Autodesk Fusion 360 part; units mm, degrees
note: some values were not read from the file. Chosen so that the rebuilt part matches the saved one: a direction. Set by a fixed rule: which sketch regions a step uses.
(part 2 of 5)
  arc A27 (-12.0685, 25.5855) -> (-12.156, 25.4753) centre (-12.0566, 25.4862) ccw
  arc A28 (-12.0685, 25.5855) -> (-11.0585, 25.7494) centre (-13.5, 37.5997) ccw
  arc A29 (-10.9406, 25.6726) -> (-11.0585, 25.7494) centre (-11.0383, 25.6515) ccw
  line L14 (-10.9406, 25.6726) -> (-10.8377, 25.1964)
  spline S14 degree 5 poles (-10.8377, 25.1964) (-10.8365, 25.1908) (-10.834, 25.1798) (-10.8298, 25.1634) (-10.8235, 25.1417) (-10.8145, 25.1148) (-10.8047, 25.0882) (-10.7944, 25.0617) (-10.7839, 25.0352) (-10.7732, 25.0088) (-10.7623, 24.9824) (-10.7512, 24.9561) (-10.7398, 24.9298) (-10.7279, 24.9037) (-10.7158, 24.8777) (-10.7032, 24.8517) (-10.6904, 24.8259) (-10.6773, 24.8001) (-10.664, 24.7744) (-10.6505, 24.7488) (-10.6368, 24.7232) (-10.6229, 24.6977) (-10.6088, 24.6723) (-10.5944, 24.6469) (-10.5798, 24.6216) (-10.565, 24.5964) (-10.55, 24.5712) (-10.5348, 24.5461) (-10.5194, 24.5211) (-10.5038, 24.4961) (-10.488, 24.4712) (-10.472, 24.4464) (-10.4558, 24.4216) (-10.4395, 24.3969) (-10.423, 24.3722) (-10.4063, 24.3476) (-10.3894, 24.3231) (-10.3724, 24.2987) (-10.3551, 24.2743) (-10.3378, 24.2499) (-10.3202, 24.2257) (-10.3025, 24.2015) (-10.2846, 24.1773) (-10.2666, 24.1533) (-10.2484, 24.1292) (-10.2301, 24.1053) (-10.2116, 24.0814) (-10.1929, 24.0576) (-10.1741, 24.0338) (-10.1551, 24.0101) (-10.136, 23.9865) (-10.1167, 23.9629) (-10.0973, 23.9394) (-10.0778, 23.9159) (-10.0581, 23.8925) (-10.0382, 23.8692) (-10.0183, 23.846) (-9.9981, 23.8228) (-9.9779, 23.7996) (-9.9575, 23.7766) (-9.9369, 23.7535) (-9.9162, 23.7306) (-9.8954, 23.7077) (-9.8745, 23.6849) (-9.8534, 23.6621) (-9.8322, 23.6395) (-9.8108, 23.6168) (-9.7893, 23.5943) (-9.7677, 23.5718) (-9.746, 23.5493) (-9.7241, 23.527) (-9.7065, 23.5091) (-9.6932, 23.4958) (-9.6844, 23.4869) (-9.6799, 23.4824) knots 0 0 0 0 0 0 0.01428571 0.02857143 0.04285714 0.05714286 0.07142857 0.08571429 0.1 0.11428571 0.12857143 0.14285714 0.15714286 0.17142857 0.18571429 0.2 0.21428571 0.22857143 0.24285714 0.25714286 0.27142857 0.28571429 0.3 0.31428571 0.32857143 0.34285714 0.35714286 0.37142857 0.38571429 0.4 0.41428571 0.42857143 0.44285714 0.45714286 0.47142857 0.48571429 0.5 0.51428571 0.52857143 0.54285714 0.55714286 0.57142857 0.58571429 0.6 0.61428571 0.62857143 0.64285714 0.65714286 0.67142857 0.68571429 0.7 0.71428571 0.72857143 0.74285714 0.75714286 0.77142857 0.78571429 0.8 0.81428571 0.82857143 0.84285714 0.85714286 0.87142857 0.88571429 0.9 0.91428571 0.92857143 0.94285714 0.95714286 0.97142857 0.98571429 1 1 1 1 1 1
  arc A30 (-9.6799, 23.4824) -> (-8.909, 23.714) centre (-13.5, 37.5997) ccw
  spline S15 degree 5 poles (-8.909, 23.714) (-8.9078, 23.7201) (-8.9053, 23.7324) (-8.9016, 23.7509) (-8.8967, 23.7755) (-8.8908, 23.8062) (-8.885, 23.8369) (-8.8794, 23.8676) (-8.8739, 23.8982) (-8.8685, 23.9289) (-8.8633, 23.9595) (-8.8583, 23.9901) (-8.8533, 24.0207) (-8.8486, 24.0513) (-8.844, 24.0818) (-8.8395, 24.1123) (-8.8352, 24.1428) (-8.831, 24.1733) (-8.827, 24.2038) (-8.8231, 24.2342) (-8.8194, 24.2646) (-8.8159, 24.295) (-8.8125, 24.3253) (-8.8092, 24.3556) (-8.8062, 24.3859) (-8.8032, 24.4162) (-8.8005, 24.4464) (-8.7979, 24.4766) (-8.7954, 24.5068) (-8.7931, 24.5369) (-8.791, 24.567) (-8.7891, 24.597) (-8.7873, 24.6271) (-8.7857, 24.6571) (-8.7842, 24.687) (-8.783, 24.7169) (-8.7819, 24.7468) (-8.7809, 24.7767) (-8.7802, 24.8065) (-8.7796, 24.8362) (-8.7792, 24.8659) (-8.779, 24.8956) (-8.779, 24.9252) (-8.7792, 24.9548) (-8.7795, 24.9843) (-8.7801, 25.0138) (-8.7808, 25.0433) (-8.7818, 25.0726) (-8.7829, 25.102) (-8.7842, 25.1312) (-8.7857, 25.1605) (-8.7875, 25.1896) (-8.7895, 25.2187) (-8.7917, 25.2477) (-8.7942, 25.2767) (-8.7968, 25.3056) (-8.7997, 25.3344) (-8.8028, 25.3632) (-8.806, 25.3919) (-8.8096, 25.4205) (-8.8134, 25.4491) (-8.8176, 25.4775) (-8.8221, 25.5058) (-8.827, 25.534) (-8.8323, 25.5621) (-8.8377, 25.5901) (-8.8433, 25.6181) (-8.8491, 25.646) (-8.8552, 25.6737) (-8.8617, 25.7014) (-8.869, 25.7287) (-8.8757, 25.7503) (-8.8812, 25.7663) (-8.8852, 25.7769) (-8.8873, 25.7822) knots -1 -1 -1 -1 -1 -1 -0.98571429 -0.97142857 -0.95714286 -0.94285714 -0.92857143 -0.91428571 -0.9 -0.88571429 -0.87142857 -0.85714286 -0.84285714 -0.82857143 -0.81428571 -0.8 -0.78571429 -0.77142857 -0.75714286 -0.74285714 -0.72857143 -0.71428571 -0.7 -0.68571429 -0.67142857 -0.65714286 -0.64285714 -0.62857143 -0.61428571 -0.6 -0.58571429 -0.57142857 -0.55714286 -0.54285714 -0.52857143 -0.51428571 -0.5 -0.48571429 -0.47142857 -0.45714286 -0.44285714 -0.42857143 -0.41428571 -0.4 -0.38571429 -0.37142857 -0.35714286 -0.34285714 -0.32857143 -0.31428571 -0.3 -0.28571429 -0.27142857 -0.25714286 -0.24285714 -0.22857143 -0.21428571 -0.2 -0.18571429 -0.17142857 -0.15714286 -0.14285714 -0.12857143 -0.11428571 -0.1 -0.08571429 -0.07142857 -0.05714286 -0.04285714 -0.02857143 -0.01428571 0 0 0 0 0 0
  line L15 (-8.8873, 25.7822) -> (-9.0638, 26.2363)
  arc A31 (-9.0077, 26.3654) -> (-9.0638, 26.2363) centre (-8.9706, 26.2725) ccw
  arc A32 (-9.0077, 26.3654) -> (-8.0746, 26.7851) centre (-13.5, 37.5997) ccw
  arc A33 (-7.9408, 26.7414) -> (-8.0746, 26.7851) centre (-8.0298, 26.6957) ccw
  line L16 (-7.9408, 26.7414) -> (-7.7182, 26.3081)
  spline S16 degree 5 poles (-7.7182, 26.3081) (-7.7156, 26.303) (-7.7103, 26.293) (-7.702, 26.2782) (-7.6903, 26.2589) (-7.6746, 26.2353) (-7.6583, 26.2121) (-7.6416, 26.1891) (-7.6245, 26.1663) (-7.6074, 26.1435) (-7.59, 26.1209) (-7.5724, 26.0983) (-7.5546, 26.076) (-7.5364, 26.0538) (-7.5179, 26.0318) (-7.4991, 26.01) (-7.48, 25.9883) (-7.4607, 25.9668) (-7.4413, 25.9454) (-7.4216, 25.9242) (-7.4017, 25.903) (-7.3817, 25.882) (-7.3614, 25.861) (-7.341, 25.8403) (-7.3203, 25.8196) (-7.2995, 25.7991) (-7.2785, 25.7786) (-7.2573, 25.7583) (-7.2359, 25.7382) (-7.2144, 25.7181) (-7.1927, 25.6981) (-7.1708, 25.6782) (-7.1488, 25.6585) (-7.1266, 25.6389) (-7.1043, 25.6193) (-7.0818, 25.5999) (-7.0592, 25.5806) (-7.0364, 25.5614) (-7.0134, 25.5423) (-6.9903, 25.5233) (-6.9671, 25.5044) (-6.9437, 25.4856) (-6.9202, 25.4669) (-6.8966, 25.4483) (-6.8728, 25.4298) (-6.8489, 25.4114) (-6.8248, 25.3931) (-6.8006, 25.375) (-6.7763, 25.3569) (-6.7518, 25.3389) (-6.7273, 25.321) (-6.7026, 25.3032) (-6.6777, 25.2855) (-6.6528, 25.2679) (-6.6277, 25.2504) (-6.6025, 25.233) (-6.5772, 25.2157) (-6.5517, 25.1985) (-6.5262, 25.1814) (-6.5005, 25.1644) (-6.4747, 25.1475) (-6.4488, 25.1307) (-6.4227, 25.114) (-6.3966, 25.0974) (-6.3703, 25.0809) (-6.3439, 25.0644) (-6.3175, 25.0481) (-6.2909, 25.0319) (-6.2642, 25.0158) (-6.2374, 24.9997) (-6.2104, 24.9838) (-6.1888, 24.9711) (-6.1726, 24.9616) (-6.1617, 24.9553) (-6.1563, 24.9522) knots 0 0 0 0 0 0 0.01428571 0.02857143 0.04285714 0.05714286 0.07142857 0.08571429 0.1 0.11428571 0.12857143 0.14285714 0.15714286 0.17142857 0.18571429 0.2 0.21428571 0.22857143 0.24285714 0.25714286 0.27142857 0.28571429 0.3 0.31428571 0.32857143 0.34285714 0.35714286 0.37142857 0.38571429 0.4 0.41428571 0.42857143 0.44285714 0.45714286 0.47142857 0.48571429 0.5 0.51428571 0.52857143 0.54285714 0.55714286 0.57142857 0.58571429 0.6 0.61428571 0.62857143 0.64285714 0.65714286 0.67142857 0.68571429 0.7 0.71428571 0.72857143 0.74285714 0.75714286 0.77142857 0.78571429 0.8 0.81428571 0.82857143 0.84285714 0.85714286 0.87142857 0.88571429 0.9 0.91428571 0.92857143 0.94285714 0.95714286 0.97142857 0.98571429 1 1 1 1 1 1
  arc A34 (-6.1563, 24.9522) -> (-5.4716, 25.3754) centre (-13.5, 37.5997) ccw
  spline S17 degree 5 poles (-5.4716, 25.3754) (-5.472, 25.3816) (-5.4727, 25.3942) (-5.4739, 25.4129) (-5.4756, 25.4379) (-5.4778, 25.4691) (-5.4802, 25.5003) (-5.4827, 25.5314) (-5.4853, 25.5624) (-5.4881, 25.5934) (-5.491, 25.6244) (-5.494, 25.6552) (-5.4972, 25.6861) (-5.5005, 25.7168) (-5.5039, 25.7475) (-5.5075, 25.7781) (-5.5112, 25.8087) (-5.5151, 25.8392) (-5.5191, 25.8697) (-5.5232, 25.9001) (-5.5275, 25.9304) (-5.532, 25.9606) (-5.5365, 25.9908) (-5.5412, 26.021) (-5.5461, 26.051) (-5.5511, 26.081) (-5.5563, 26.1109) (-5.5616, 26.1407) (-5.567, 26.1705) (-5.5726, 26.2002) (-5.5784, 26.2298) (-5.5843, 26.2594) (-5.5903, 26.2888) (-5.5965, 26.3182) (-5.6029, 26.3475) (-5.6094, 26.3768) (-5.6161, 26.4059) (-5.6229, 26.435) (-5.6299, 26.464) (-5.637, 26.4929) (-5.6443, 26.5217) (-5.6518, 26.5504) (-5.6595, 26.579) (-5.6673, 26.6075) (-5.6753, 26.6359) (-5.6834, 26.6643) (-5.6918, 26.6925) (-5.7003, 26.7207) (-5.709, 26.7487) (-5.7178, 26.7766) (-5.7269, 26.8045) (-5.7361, 26.8322) (-5.7456, 26.8597) (-5.7552, 26.8872) (-5.7651, 26.9145) (-5.7751, 26.9418) (-5.7854, 26.9689) (-5.7958, 26.9959) (-5.8064, 27.0228) (-5.8172, 27.0495) (-5.8283, 27.0761) (-5.8397, 27.1024) (-5.8514, 27.1286) (-5.8634, 27.1546) (-5.8757, 27.1804) (-5.8883, 27.206) (-5.9009, 27.2316) (-5.9138, 27.257) (-5.9268, 27.2823) (-5.9403, 27.3073) (-5.9544, 27.3318) (-5.9664, 27.3509) (-5.9759, 27.365) (-5.9825, 27.3742) (-5.9858, 27.3787) knots -1 -1 -1 -1 -1 -1 -0.98571429 -0.97142857 -0.95714286 -0.94285714 -0.92857143 -0.91428571 -0.9 -0.88571429 -0.87142857 -0.85714286 -0.84285714 -0.82857143 -0.81428571 -0.8 -0.78571429 -0.77142857 -0.75714286 -0.74285714 -0.72857143 -0.71428571 -0.7 -0.68571429 -0.67142857 -0.65714286 -0.64285714 -0.62857143 -0.61428571 -0.6 -0.58571429 -0.57142857 -0.55714286 -0.54285714 -0.52857143 -0.51428571 -0.5 -0.48571429 -0.47142857 -0.45714286 -0.44285714 -0.42857143 -0.41428571 -0.4 -0.38571429 -0.37142857 -0.35714286 -0.34285714 -0.32857143 -0.31428571 -0.3 -0.28571429 -0.27142857 -0.25714286 -0.24285714 -0.22857143 -0.21428571 -0.2 -0.18571429 -0.17142857 -0.15714286 -0.14285714 -0.12857143 -0.11428571 -0.1 -0.08571429 -0.07142857 -0.05714286 -0.04285714 -0.02857143 -0.01428571 0 0 0 0 0 0
  line L17 (-5.9858, 27.3787) -> (-6.2739, 27.7717)
  arc A35 (-6.2531, 27.9109) -> (-6.2739, 27.7717) centre (-6.1932, 27.8308) ccw
  arc A36 (-6.2531, 27.9109) -> (-5.4605, 28.5578) centre (-13.5, 37.5997) ccw
  arc A37 (-5.3199, 28.5502) -> (-5.4605, 28.5578) centre (-5.394, 28.4831) ccw
  line L18 (-5.3199, 28.5502) -> (-4.9927, 28.1892)
  spline S18 degree 5 poles (-4.9927, 28.1892) (-4.9889, 28.1851) (-4.9812, 28.1768) (-4.9694, 28.1646) (-4.953, 28.149) (-4.9318, 28.1303) (-4.91, 28.1121) (-4.8879, 28.0942) (-4.8656, 28.0766) (-4.8431, 28.059) (-4.8204, 28.0416) (-4.7976, 28.0244) (-4.7746, 28.0074) (-4.7513, 27.9907) (-4.7278, 27.9742) (-4.704, 27.958) (-4.6799, 27.9421) (-4.6557, 27.9263) (-4.6313, 27.9107) (-4.6068, 27.8952) (-4.5822, 27.8799) (-4.5574, 27.8648) (-4.5324, 27.8498) (-4.5073, 27.835) (-4.482, 27.8204) (-4.4565, 27.806) (-4.431, 27.7917) (-4.4052, 27.7776) (-4.3794, 27.7636) (-4.3534, 27.7498) (-4.3272, 27.7361) (-4.301, 27.7226) (-4.2746, 27.7092) (-4.2481, 27.696) (-4.2215, 27.6829) (-4.1947, 27.6699) (-4.1678, 27.6571) (-4.1409, 27.6445) (-4.1138, 27.632) (-4.0865, 27.6196) (-4.0592, 27.6073) (-4.0318, 27.5952) (-4.0042, 27.5833) (-3.9766, 27.5714) (-3.9488, 27.5597) (-3.9209, 27.5482) (-3.893, 27.5367) (-3.8649, 27.5254) (-3.8367, 27.5143) (-3.8084, 27.5032) (-3.7801, 27.4923) (-3.7516, 27.4815) (-3.723, 27.4708) (-3.6944, 27.4603) (-3.6656, 27.4499) (-3.6368, 27.4396) (-3.6078, 27.4295) (-3.5788, 27.4195) (-3.5497, 27.4096) (-3.5205, 27.3998) (-3.4912, 27.3901) (-3.4618, 27.3806) (-3.4323, 27.3712) (-3.4028, 27.3619) (-3.3731, 27.3527) (-3.3434, 27.3437) (-3.3136, 27.3348) (-3.2837, 27.326) (-3.2538, 27.3173) (-3.2237, 27.3088) (-3.1936, 27.3003) (-3.1694, 27.2937) (-3.1513, 27.2887) (-3.1391, 27.2855) (-3.1331, 27.2838) knots 0 0 0 0 0 0 0.01428571 0.02857143 0.04285714 0.05714286 0.07142857 0.08571429 0.1 0.11428571 0.12857143 0.14285714 0.15714286 0.17142857 0.18571429 0.2 0.21428571 0.22857143 0.24285714 0.25714286 0.27142857 0.28571429 0.3 0.31428571 0.32857143 0.34285714 0.35714286 0.37142857 0.38571429 0.4 0.41428571 0.42857143 0.44285714 0.45714286 0.47142857 0.48571429 0.5 0.51428571 0.52857143 0.54285714 0.55714286 0.57142857 0.58571429 0.6 0.61428571 0.62857143 0.64285714 0.65714286 0.67142857 0.68571429 0.7 0.71428571 0.72857143 0.74285714 0.75714286 0.77142857 0.78571429 0.8 0.81428571 0.82857143 0.84285714 0.85714286 0.87142857 0.88571429 0.9 0.91428571 0.92857143 0.94285714 0.95714286 0.97142857 0.98571429 1 1 1 1 1 1
  arc A38 (-3.1331, 27.2838) -> (-2.5812, 27.8698) centre (-13.5, 37.5997) ccw
  spline S19 degree 5 poles (-2.5812, 27.8698) (-2.5832, 27.8757) (-2.5872, 27.8877) (-2.5932, 27.9055) (-2.6013, 27.9292) (-2.6115, 27.9588) (-2.6219, 27.9883) (-2.6323, 28.0177) (-2.6429, 28.047) (-2.6536, 28.0762) (-2.6644, 28.1053) (-2.6753, 28.1343) (-2.6864, 28.1633) (-2.6975, 28.1921) (-2.7088, 28.2209) (-2.7202, 28.2496) (-2.7317, 28.2781) (-2.7433, 28.3066) (-2.7551, 28.335) (-2.767, 28.3633) (-2.7789, 28.3914) (-2.7911, 28.4195) (-2.8033, 28.4475) (-2.8156, 28.4754) (-2.8281, 28.5031) (-2.8407, 28.5308) (-2.8534, 28.5584) (-2.8663, 28.5858) (-2.8792, 28.6132) (-2.8923, 28.6404) (-2.9055, 28.6675) (-2.9189, 28.6945) (-2.9324, 28.7214) (-2.946, 28.7482) (-2.9597, 28.7749) (-2.9735, 28.8014) (-2.9875, 28.8278) (-3.0017, 28.8542) (-3.0159, 28.8803) (-3.0303, 28.9064) (-3.0448, 28.9323) (-3.0595, 28.9581) (-3.0743, 28.9838) (-3.0892, 29.0093) (-3.1043, 29.0347) (-3.1195, 29.06) (-3.1348, 29.0851) (-3.1503, 29.1101) (-3.166, 29.1349) (-3.1818, 29.1596) (-3.1977, 29.1841) (-3.2138, 29.2085) (-3.2301, 29.2327) (-3.2465, 29.2567) (-3.2631, 29.2806) (-3.2799, 29.3043) (-3.2968, 29.3278) (-3.3138, 29.3512) (-3.331, 29.3744) (-3.3484, 29.3974) (-3.366, 29.4202) (-3.3838, 29.4428) (-3.4019, 29.465) (-3.4202, 29.487) (-3.4388, 29.5087) (-3.4575, 29.5303) (-3.4764, 29.5516) (-3.4954, 29.5729) (-3.5145, 29.5939) (-3.534, 29.6146) (-3.554, 29.6346) (-3.5705, 29.65) (-3.5834, 29.6611) (-3.5921, 29.6683) (-3.5965, 29.6718) knots -1 -1 -1 -1 -1 -1 -0.98571429 -0.97142857 -0.95714286 -0.94285714 -0.92857143 -0.91428571 -0.9 -0.88571429 -0.87142857 -0.85714286 -0.84285714 -0.82857143 -0.81428571 -0.8 -0.78571429 -0.77142857 -0.75714286 -0.74285714 -0.72857143 -0.71428571 -0.7 -0.68571429 -0.67142857 -0.65714286 -0.64285714 -0.62857143 -0.61428571 -0.6 -0.58571429 -0.57142857 -0.55714286 -0.54285714 -0.52857143 -0.51428571 -0.5 -0.48571429 -0.47142857 -0.45714286 -0.44285714 -0.42857143 -0.41428571 -0.4 -0.38571429 -0.37142857 -0.35714286 -0.34285714 -0.32857143 -0.31428571 -0.3 -0.28571429 -0.27142857 -0.25714286 -0.24285714 -0.22857143 -0.21428571 -0.2 -0.18571429 -0.17142857 -0.15714286 -0.14285714 -0.12857143 -0.11428571 -0.1 -0.08571429 -0.07142857 -0.05714286 -0.04285714 -0.02857143 -0.01428571 0 0 0 0 0 0
  line L19 (-3.5965, 29.6718) -> (-3.9764, 29.9768)
  arc A39 (-3.9924, 30.1166) -> (-3.9764, 29.9768) centre (-3.9138, 30.0548) ccw
  arc A40 (-3.9924, 30.1166) -> (-3.3942, 30.9467) centre (-13.5, 37.5997) ccw
  arc A41 (-3.2565, 30.9757) -> (-3.3942, 30.9467) centre (-3.3107, 30.8917) ccw
  line L20 (-3.2565, 30.9757) -> (-2.847, 30.7117)
  spline S20 degree 5 poles (-2.847, 30.7117) (-2.8422, 30.7087) (-2.8327, 30.7027) (-2.8181, 30.694) (-2.7982, 30.6832) (-2.7729, 30.6705) (-2.7471, 30.6586) (-2.7211, 30.6471) (-2.695, 30.6358) (-2.6687, 30.6247) (-2.6424, 30.6137) (-2.6159, 30.603) (-2.5893, 30.5925) (-2.5624, 30.5824) (-2.5354, 30.5726) (-2.5082, 30.5631) (-2.4809, 30.5539) (-2.4534, 30.545) (-2.4258, 30.5362) (-2.3982, 30.5276) (-2.3704, 30.5192) (-2.3425, 30.511) (-2.3145, 30.503) (-2.2864, 30.4952) (-2.2582, 30.4877) (-2.2299, 30.4803) (-2.2015, 30.4731) (-2.173, 30.4661) (-2.1444, 30.4593) (-2.1157, 30.4527) (-2.0869, 30.4463) (-2.058, 30.44) (-2.0291, 30.4339) (-2.0001, 30.428) (-1.971, 30.4222) (-1.9418, 30.4167) (-1.9125, 30.4113) (-1.8832, 30.406) (-1.8537, 30.401) (-1.8242, 30.396) (-1.7947, 30.3913) (-1.765, 30.3867) (-1.7353, 30.3823) (-1.7056, 30.378) (-1.6757, 30.3739) (-1.6458, 30.3699) (-1.6158, 30.3661) (-1.5858, 30.3624) (-1.5557, 30.3589) (-1.5255, 30.3556) (-1.4953, 30.3524) (-1.465, 30.3493) (-1.4346, 30.3464) (-1.4042, 30.3437) (-1.3738, 30.3411) (-1.3432, 30.3386) (-1.3127, 30.3363) (-1.282, 30.3341) (-1.2513, 30.3321) (-1.2206, 30.3302) (-1.1898, 30.3285) (-1.1589, 30.3269) (-1.128, 30.3254) (-1.0971, 30.3241) (-1.0661, 30.3229) (-1.035, 30.3219) (-1.0039, 30.321) (-0.9728, 30.3202) (-0.9416, 30.3196) (-0.9104, 30.3191) (-0.8791, 30.3188) (-0.854, 30.3186) (-0.8352, 30.3185) (-0.8226, 30.3185) (-0.8164, 30.3185) knots 0 0 0 0 0 0 0.01428571 0.02857143 0.04285714 0.05714286 0.07142857 0.08571429 0.1 0.11428571 0.12857143 0.14285714 0.15714286 0.17142857 0.18571429 0.2 0.21428571 0.22857143 0.24285714 0.25714286 0.27142857 0.28571429 0.3 0.31428571 0.32857143 0.34285714 0.35714286 0.37142857 0.38571429 0.4 0.41428571 0.42857143 0.44285714 0.45714286 0.47142857 0.48571429 0.5 0.51428571 0.52857143 0.54285714 0.55714286 0.57142857 0.58571429 0.6 0.61428571 0.62857143 0.64285714 0.65714286 0.67142857 0.68571429 0.7 0.71428571 0.72857143 0.74285714 0.75714286 0.77142857 0.78571429 0.8 0.81428571 0.82857143 0.84285714 0.85714286 0.87142857 0.88571429 0.9 0.91428571 0.92857143 0.94285714 0.95714286 0.97142857 0.98571429 1 1 1 1 1 1
  arc A42 (-0.8164, 30.3185) -> (-0.435, 31.0273) centre (-13.5, 37.5997) ccw
  spline S21 degree 5 poles (-0.435, 31.0273) (-0.4385, 31.0326) (-0.4454, 31.043) (-0.4558, 31.0587) (-0.4698, 31.0795) (-0.4873, 31.1054) (-0.5049, 31.1312) (-0.5226, 31.1569) (-0.5404, 31.1825) (-0.5583, 31.2079) (-0.5763, 31.2333) (-0.5944, 31.2585) (-0.6125, 31.2836) (-0.6308, 31.3086) (-0.6491, 31.3334) (-0.6675, 31.3582) (-0.686, 31.3828) (-0.7046, 31.4073) (-0.7233, 31.4317) (-0.7421, 31.4559) (-0.761, 31.48) (-0.7799, 31.504) (-0.799, 31.5279) (-0.8181, 31.5516) (-0.8374, 31.5752) (-0.8567, 31.5987) (-0.8761, 31.622) (-0.8956, 31.6452) (-0.9152, 31.6682) (-0.9349, 31.6911) (-0.9547, 31.7139) (-0.9746, 31.7366) (-0.9946, 31.7591) (-1.0146, 31.7814) (-1.0348, 31.8036) (-1.0551, 31.8257) (-1.0754, 31.8476) (-1.0959, 31.8693) (-1.1164, 31.8909) (-1.137, 31.9124) (-1.1578, 31.9337) (-1.1786, 31.9548) (-1.1995, 31.9757) (-1.2206, 31.9965) (-1.2417, 32.0172) (-1.2629, 32.0376) (-1.2843, 32.0579) (-1.3057, 32.078) (-1.3272, 32.098) (-1.3489, 32.1177) (-1.3706, 32.1373) (-1.3925, 32.1567) (-1.4145, 32.1758) (-1.4366, 32.1948) (-1.4588, 32.2135) (-1.4811, 32.2321) (-1.5035, 32.2505) (-1.526, 32.2686) (-1.5486, 32.2866) (-1.5714, 32.3044) (-1.5943, 32.3218) (-1.6173, 32.339) (-1.6406, 32.3558) (-1.664, 32.3723) (-1.6875, 32.3884) (-1.7112, 32.4044) (-1.7349, 32.4202) (-1.7588, 32.4358) (-1.7827, 32.4511) (-1.8068, 32.4661) (-1.8313, 32.4802) (-1.8513, 32.4908) (-1.8666, 32.4982) (-1.8769, 32.5029) (-1.8821, 32.5052) knots -1 -1 -1 -1 -1 -1 -0.98571429 -0.97142857 -0.95714286 -0.94285714 -0.92857143 -0.91428571 -0.9 -0.88571429 -0.87142857 -0.85714286 -0.84285714 -0.82857143 -0.81428571 -0.8 -0.78571429 -0.77142857 -0.75714286 -0.74285714 -0.72857143 -0.71428571 -0.7 -0.68571429 -0.67142857 -0.65714286 -0.64285714 -0.62857143 -0.61428571 -0.6 -0.58571429 -0.57142857 -0.55714286 -0.54285714 -0.52857143 -0.51428571 -0.5 -0.48571429 -0.47142857 -0.45714286 -0.44285714 -0.42857143 -0.41428571 -0.4 -0.38571429 -0.37142857 -0.35714286 -0.34285714 -0.32857143 -0.31428571 -0.3 -0.28571429 -0.27142857 -0.25714286 -0.24285714 -0.22857143 -0.21428571 -0.2 -0.18571429 -0.17142857 -0.15714286 -0.14285714 -0.12857143 -0.11428571 -0.1 -0.08571429 -0.07142857 -0.05714286 -0.04285714 -0.02857143 -0.01428571 0 0 0 0 0 0
  line L21 (-1.8821, 32.5052) -> (-2.328, 32.7014)
  arc A43 (-2.3796, 32.8324) -> (-2.328, 32.7014) centre (-2.2877, 32.793) ccw
  arc A44 (-2.3796, 32.8324) -> (-2.0166, 33.7889) centre (-13.5, 37.5997) ccw
  arc A45 (-1.8911, 33.8527) -> (-2.0166, 33.7889) centre (-1.9217, 33.7575) ccw
  line L22 (-1.8911, 33.8527) -> (-1.4272, 33.7037)
  spline S22 degree 5 poles (-1.4272, 33.7037) (-1.4219, 33.7019) (-1.411, 33.6986) (-1.3947, 33.694) (-1.3728, 33.6887) (-1.345, 33.683) (-1.317, 33.6782) (-1.289, 33.6738) (-1.2608, 33.6696) (-1.2325, 33.6657) (-1.2042, 33.6619) (-1.1759, 33.6584) (-1.1474, 33.6552) (-1.1189, 33.6524) (-1.0903, 33.6499) (-1.0616, 33.6478) (-1.0328, 33.646) (-1.0039, 33.6444) (-0.975, 33.6431) (-0.946, 33.642) (-0.917, 33.641) (-0.888, 33.6403) (-0.8589, 33.6398) (-0.8297, 33.6396) (-0.8005, 33.6396) (-0.7713, 33.6398) (-0.742, 33.6402) (-0.7126, 33.6409) (-0.6832, 33.6417) (-0.6538, 33.6427) (-0.6243, 33.644) (-0.5949, 33.6454) (-0.5653, 33.647) (-0.5357, 33.6488) (-0.5061, 33.6507) (-0.4765, 33.6529) (-0.4468, 33.6553) (-0.4171, 33.6578) (-0.3874, 33.6605) (-0.3576, 33.6634) (-0.3279, 33.6665) (-0.298, 33.6697) (-0.2682, 33.6731) (-0.2383, 33.6767) (-0.2084, 33.6804) (-0.1785, 33.6844) (-0.1486, 33.6884) (-0.1186, 33.6927) (-0.0886, 33.6971) (-0.0586, 33.7017) (-0.0286, 33.7064) (0.0015, 33.7113) (0.0315, 33.7163) (0.0616, 33.7215) (0.0917, 33.7269) (0.1218, 33.7324) (0.152, 33.7381) (0.1821, 33.7439) (0.2123, 33.7499) (0.2425, 33.7561) (0.2727, 33.7624) (0.3029, 33.7688) (0.3331, 33.7754) (0.3634, 33.7821) (0.3936, 33.789) (0.4239, 33.796) (0.4541, 33.8032) (0.4844, 33.8105) (0.5147, 33.818) (0.545, 33.8256) (0.5753, 33.8334) (0.5996, 33.8397) (0.6178, 33.8445) (0.6299, 33.8477) (0.636, 33.8494) knots 0 0 0 0 0 0 0.01428571 0.02857143 0.04285714 0.05714286 0.07142857 0.08571429 0.1 0.11428571 0.12857143 0.14285714 0.15714286 0.17142857 0.18571429 0.2 0.21428571 0.22857143 0.24285714 0.25714286 0.27142857 0.28571429 0.3 0.31428571 0.32857143 0.34285714 0.35714286 0.37142857 0.38571429 0.4 0.41428571 0.42857143 0.44285714 0.45714286 0.47142857 0.48571429 0.5 0.51428571 0.52857143 0.54285714 0.55714286 0.57142857 0.58571429 0.6 0.61428571 0.62857143 0.64285714 0.65714286 0.67142857 0.68571429 0.7 0.71428571 0.72857143 0.74285714 0.75714286 0.77142857 0.78571429 0.8 0.81428571 0.82857143 0.84285714 0.85714286 0.87142857 0.88571429 0.9 0.91428571 0.92857143 0.94285714 0.95714286 0.97142857 0.98571429 1 1 1 1 1 1
  arc A46 (0.636, 33.8494) -> (0.8209, 34.6327) centre (-13.5, 37.5997) ccw
  spline S23 degree 5 poles (0.8209, 34.6327) (0.8162, 34.6369) (0.8068, 34.6452) (0.7927, 34.6577) (0.7738, 34.6742) (0.7501, 34.6946) (0.7264, 34.715) (0.7027, 34.7352) (0.6789, 34.7553) (0.655, 34.7753) (0.6311, 34.7951) (0.6071, 34.8148) (0.5831, 34.8343) (0.559, 34.8538) (0.5349, 34.873) (0.5107, 34.8921) (0.4864, 34.9111) (0.4621, 34.93) (0.4377, 34.9487) (0.4133, 34.9672) (0.3888, 34.9856) (0.3643, 35.0039) (0.3397, 35.022) (0.3151, 35.04) (0.2904, 35.0578) (0.2657, 35.0755) (0.2409, 35.093) (0.216, 35.1103) (0.1911, 35.1275) (0.1662, 35.1446) (0.1412, 35.1614) (0.1161, 35.1782) (0.091, 35.1947) (0.0658, 35.2111) (0.0406, 35.2273) (0.0153, 35.2434) (-0.01, 35.2593) (-0.0354, 35.275) (-0.0608, 35.2906) (-0.0863, 35.3059) (-0.1118, 35.3211) (-0.1374, 35.3361) (-0.1631, 35.351) (-0.1888, 35.3656) (-0.2145, 35.3801) (-0.2403, 35.3943) (-0.2662, 35.4084) (-0.2921, 35.4223) (-0.3181, 35.436) (-0.3441, 35.4495) (-0.3702, 35.4628) (-0.3963, 35.4758) (-0.4225, 35.4886) (-0.4487, 35.5012) (-0.475, 35.5136) (-0.5014, 35.5257) (-0.5278, 35.5376) (-0.5542, 35.5494) (-0.5807, 35.5609) (-0.6073, 35.5721) (-0.6339, 35.5831) (-0.6606, 35.5937) (-0.6874, 35.6039) (-0.7143, 35.6138) (-0.7413, 35.6233) (-0.7682, 35.6326) (-0.7953, 35.6417) (-0.8223, 35.6506) (-0.8494, 35.6592) (-0.8766, 35.6674) (-0.9039, 35.6748) (-0.926, 35.6798) (-0.9426, 35.683) (-0.9538, 35.6848) (-0.9594, 35.6857) knots -1 -1 -1 -1 -1 -1 -0.98571429 -0.97142857 -0.95714286 -0.94285714 -0.92857143 -0.91428571 -0.9 -0.88571429 -0.87142857 -0.85714286 -0.84285714 -0.82857143 -0.81428571 -0.8 -0.78571429 -0.77142857 -0.75714286 -0.74285714 -0.72857143 -0.71428571 -0.7 -0.68571429 -0.67142857 -0.65714286 -0.64285714 -0.62857143 -0.61428571 -0.6 -0.58571429 -0.57142857 -0.55714286 -0.54285714 -0.52857143 -0.51428571 -0.5 -0.48571429 -0.47142857 -0.45714286 -0.44285714 -0.42857143 -0.41428571 -0.4 -0.38571429 -0.37142857 -0.35714286 -0.34285714 -0.32857143 -0.31428571 -0.3 -0.28571429 -0.27142857 -0.25714286 -0.24285714 -0.22857143 -0.21428571 -0.2 -0.18571429 -0.17142857 -0.15714286 -0.14285714 -0.12857143 -0.11428571 -0.1 -0.08571429 -0.07142857 -0.05714286 -0.04285714 -0.02857143 -0.01428571 0 0 0 0 0 0
  line L23 (-0.9594, 35.6857) -> (-1.4409, 35.7599)
  arc A47 (-1.5247, 35.873) -> (-1.4409, 35.7599) centre (-1.4257, 35.8587) ccw
  arc A48 (-1.5247, 35.873) -> (-1.4216, 36.8909) centre (-13.5, 37.5997) ccw
  arc A49 (-1.3169, 36.9849) -> (-1.4216, 36.8909) centre (-1.3218, 36.8851) ccw
  line L24 (-1.3169, 36.9849) -> (-0.8302, 36.9611)
  spline S24 degree 5 poles (-0.8302, 36.9611) (-0.8246, 36.9608) (-0.8133, 36.9604) (-0.7963, 36.9602) (-0.7737, 36.9607) (-0.7455, 36.9624) (-0.7172, 36.965) (-0.6889, 36.968) (-0.6606, 36.9713) (-0.6323, 36.9748) (-0.604, 36.9785) (-0.5757, 36.9824) (-0.5474, 36.9867) (-0.5191, 36.9913) (-0.4908, 36.9964) (-0.4625, 37.0018) (-0.4343, 37.0075) (-0.406, 37.0134) (-0.3777, 37.0196) (-0.3495, 37.026) (-0.3212, 37.0326) (-0.293, 37.0395) (-0.2647, 37.0465) (-0.2365, 37.0538) (-0.2083, 37.0614) (-0.1801, 37.0692) (-0.1519, 37.0772) (-0.1237, 37.0854) (-0.0955, 37.0938) (-0.0674, 37.1024) (-0.0392, 37.1112) (-0.0111, 37.1202) (0.017, 37.1294) (0.0451, 37.1388) (0.0732, 37.1484) (0.1012, 37.1581) (0.1293, 37.1681) (0.1573, 37.1782) (0.1853, 37.1885) (0.2133, 37.199) (0.2413, 37.2097) (0.2693, 37.2205) (0.2972, 37.2316) (0.3251, 37.2427) (0.3531, 37.2541) (0.3809, 37.2656) (0.4088, 37.2773) (0.4366, 37.2892) (0.4645, 37.3012) (0.4923, 37.3134) (0.5201, 37.3257) (0.5478, 37.3382) (0.5755, 37.3509) (0.6033, 37.3637) (0.6309, 37.3767) (0.6586, 37.3898) (0.6863, 37.4031) (0.7139, 37.4165) (0.7415, 37.4301) (0.769, 37.4438) (0.7966, 37.4577) (0.8241, 37.4718) (0.8516, 37.486) (0.879, 37.5003) (0.9065, 37.5148) (0.9339, 37.5294) (0.9613, 37.5442) (0.9886, 37.5591) (1.0159, 37.5741) (1.0432, 37.5893) (1.0705, 37.6047) (1.0923, 37.6171) (1.1086, 37.6264) (1.1195, 37.6327) (1.125, 37.6358) knots 0 0 0 0 0 0 0.01428571 0.02857143 0.04285714 0.05714286 0.07142857 0.08571429 0.1 0.11428571 0.12857143 0.14285714 0.15714286 0.17142857 0.18571429 0.2 0.21428571 0.22857143 0.24285714 0.25714286 0.27142857 0.28571429 0.3 0.31428571 0.32857143 0.34285714 0.35714286 0.37142857 0.38571429 0.4 0.41428571 0.42857143 0.44285714 0.45714286 0.47142857 0.48571429 0.5 0.51428571 0.52857143 0.54285714 0.55714286 0.57142857 0.58571429 0.6 0.61428571 0.62857143 0.64285714 0.65714286 0.67142857 0.68571429 0.7 0.71428571 0.72857143 0.74285714 0.75714286 0.77142857 0.78571429 0.8 0.81428571 0.82857143 0.84285714 0.85714286 0.87142857 0.88571429 0.9 0.91428571 0.92857143 0.94285714 0.95714286 0.97142857 0.98571429 1 1 1 1 1 1
  arc A50 (1.125, 37.6358) -> (1.1008, 38.4403) centre (-13.5, 37.5997) ccw
  spline S25 degree 5 poles (1.1008, 38.4403) (1.0952, 38.4432) (1.084, 38.4488) (1.0671, 38.4571) (1.0446, 38.4682) (1.0165, 38.4818) (0.9883, 38.4954) (0.9601, 38.5088) (0.9319, 38.522) (0.9037, 38.5351) (0.8755, 38.5481) (0.8472, 38.5609) (0.819, 38.5735) (0.7907, 38.5861) (0.7624, 38.5984) (0.734, 38.6106) (0.7057, 38.6227) (0.6773, 38.6346) (0.649, 38.6464) (0.6206, 38.658) (0.5922, 38.6694) (0.5637, 38.6807) (0.5353, 38.6918) (0.5069, 38.7028) (0.4784, 38.7136) (0.4499, 38.7243) (0.4215, 38.7348) (0.393, 38.7451) (0.3645, 38.7553) (0.336, 38.7653) (0.3074, 38.7751) (0.2789, 38.7848) (0.2503, 38.7943) (0.2218, 38.8036) (0.1932, 38.8127) (0.1647, 38.8217) (0.1361, 38.8305) (0.1075, 38.8391) (0.0789, 38.8476) (0.0503, 38.8558) (0.0217, 38.8639) (-0.0069, 38.8718) (-0.0355, 38.8794) (-0.0641, 38.8869) (-0.0927, 38.8942) (-0.1214, 38.9013) (-0.15, 38.9082) (-0.1786, 38.9149) (-0.2072, 38.9214) (-0.2358, 38.9277) (-0.2645, 38.9338) (-0.2931, 38.9397) (-0.3217, 38.9453) (-0.3503, 38.9506) (-0.3789, 38.9558) (-0.4075, 38.9607) (-0.4361, 38.9654) (-0.4647, 38.9699) (-0.4933, 38.9741) (-0.5218, 38.9781) (-0.5504, 38.9818) (-0.5789, 38.9851) (-0.6075, 38.9881) (-0.636, 38.9906) (-0.6645, 38.9928) (-0.6929, 38.9948) (-0.7214, 38.9966) (-0.7498, 38.9982) (-0.7782, 38.9996) (-0.8066, 39.0004) (-0.8349, 39.0005) (-0.8575, 38.9996) (-0.8744, 38.9984) (-0.8857, 38.9973) (-0.8913, 38.9967) knots -1 -1 -1 -1 -1 -1 -0.98571429 -0.97142857 -0.95714286 -0.94285714 -0.92857143 -0.91428571 -0.9 -0.88571429 -0.87142857 -0.85714286 -0.84285714 -0.82857143 -0.81428571 -0.8 -0.78571429 -0.77142857 -0.75714286 -0.74285714 -0.72857143 -0.71428571 -0.7 -0.68571429 -0.67142857 -0.65714286 -0.64285714 -0.62857143 -0.61428571 -0.6 -0.58571429 -0.57142857 -0.55714286 -0.54285714 -0.52857143 -0.51428571 -0.5 -0.48571429 -0.47142857 -0.45714286 -0.44285714 -0.42857143 -0.41428571 -0.4 -0.38571429 -0.37142857 -0.35714286 -0.34285714 -0.32857143 -0.31428571 -0.3 -0.28571429 -0.27142857 -0.25714286 -0.24285714 -0.22857143 -0.21428571 -0.2 -0.18571429 -0.17142857 -0.15714286 -0.14285714 -0.12857143 -0.11428571 -0.1 -0.08571429 -0.07142857 -0.05714286 -0.04285714 -0.02857143 -0.01428571 0 0 0 0 0 0
  line L25 (-0.8913, 38.9967) -> (-1.3756, 38.9437)
  arc A51 (-1.4858, 39.0313) -> (-1.3756, 38.9437) centre (-1.3865, 39.0431) ccw
  arc A52 (-1.4858, 39.0313) -> (-1.6497, 40.0412) centre (-13.5, 37.5997) ccw
  arc A53 (-1.5729, 40.1591) -> (-1.6497, 40.0412) centre (-1.5517, 40.0614) ccw
  line L26 (-1.5729, 40.1591) -> (-1.0967, 40.262)
  spline S26 degree 5 poles (-1.0967, 40.262) (-1.0911, 40.2632) (-1.0801, 40.2657) (-1.0637, 40.2699) (-1.042, 40.2763) (-1.0151, 40.2853) (-0.9885, 40.295) (-0.9619, 40.3053) (-0.9355, 40.3158) (-0.9091, 40.3265) (-0.8827, 40.3374) (-0.8563, 40.3485) (-0.8301, 40.36) (-0.804, 40.3718) (-0.778, 40.384) (-0.752, 40.3965) (-0.7262, 40.4093) (-0.7004, 40.4224) (-0.6747, 40.4357) (-0.6491, 40.4492) (-0.6235, 40.4629) (-0.598, 40.4768) (-0.5725, 40.4909) (-0.5472, 40.5053) (-0.5219, 40.5199) (-0.4966, 40.5347) (-0.4715, 40.5497) (-0.4464, 40.5649) (-0.4213, 40.5804) (-0.3964, 40.596) (-0.3715, 40.6118) (-0.3466, 40.6277) (-0.3219, 40.6439) (-0.2972, 40.6602) (-0.2725, 40.6767) (-0.2479, 40.6934) (-0.2234, 40.7103) (-0.1989, 40.7274) (-0.1746, 40.7446) (-0.1502, 40.762) (-0.126, 40.7795) (-0.1018, 40.7972) (-0.0776, 40.8151) (-0.0535, 40.8331) (-0.0295, 40.8513) (-0.0056, 40.8697) (0.0183, 40.8882) (0.0421, 40.9068) (0.0659, 40.9256) (0.0896, 40.9446) (0.1132, 40.9637) (0.1368, 40.983) (0.1603, 41.0024) (0.1838, 41.0219) (0.2072, 41.0416) (0.2305, 41.0615) (0.2538, 41.0815) (0.277, 41.1016) (0.3001, 41.1219) (0.3232, 41.1423) (0.3462, 41.1628) (0.3691, 41.1835) (0.392, 41.2043) (0.4148, 41.2253) (0.4376, 41.2463) (0.4603, 41.2676) (0.4829, 41.2889) (0.5054, 41.3104) (0.5279, 41.332) (0.5504, 41.3538) (0.5727, 41.3756) (0.5906, 41.3932) (0.6039, 41.4065) (0.6128, 41.4154) (0.6173, 41.4198) knots 0 0 0 0 0 0 0.01428571 0.02857143 0.04285714 0.05714286 0.07142857 0.08571429 0.1 0.11428571 0.12857143 0.14285714 0.15714286 0.17142857 0.18571429 0.2 0.21428571 0.22857143 0.24285714 0.25714286 0.27142857 0.28571429 0.3 0.31428571 0.32857143 0.34285714 0.35714286 0.37142857 0.38571429 0.4 0.41428571 0.42857143 0.44285714 0.45714286 0.47142857 0.48571429 0.5 0.51428571 0.52857143 0.54285714 0.55714286 0.57142857 0.58571429 0.6 0.61428571 0.62857143 0.64285714 0.65714286 0.67142857 0.68571429 0.7 0.71428571 0.72857143 0.74285714 0.75714286 0.77142857 0.78571429 0.8 0.81428571 0.82857143 0.84285714 0.85714286 0.87142857 0.88571429 0.9 0.91428571 0.92857143 0.94285714 0.95714286 0.97142857 0.98571429 1 1 1 1 1 1
  arc A54 (0.6173, 41.4198) -> (0.3857, 42.1907) centre (-13.5, 37.5997) ccw
  spline S27 degree 5 poles (0.3857, 42.1907) (0.3796, 42.1919) (0.3673, 42.1944) (0.3488, 42.1981) (0.3242, 42.203) (0.2935, 42.2089) (0.2628, 42.2147) (0.2321, 42.2204) (0.2015, 42.2258) (0.1708, 42.2312) (0.1402, 42.2364) (0.1096, 42.2415) (0.079, 42.2464) (0.0484, 42.2511) (0.0179, 42.2558) (-0.0126, 42.2602) (-0.0431, 42.2645) (-0.0736, 42.2687) (-0.104, 42.2727) (-0.1345, 42.2766) (-0.1649, 42.2803) (-0.1952, 42.2838) (-0.2256, 42.2872) (-0.2559, 42.2905) (-0.2862, 42.2936) (-0.3164, 42.2965) (-0.3467, 42.2992) (-0.3769, 42.3019) (-0.407, 42.3043) (-0.4372, 42.3066) (-0.4673, 42.3087) (-0.4973, 42.3106) (-0.5274, 42.3124) (-0.5574, 42.314) (-0.5873, 42.3155) (-0.6172, 42.3167) (-0.6471, 42.3178) (-0.6769, 42.3188) (-0.7067, 42.3195) (-0.7365, 42.3201) (-0.7662, 42.3205) (-0.7959, 42.3207) (-0.8255, 42.3207) (-0.8551, 42.3205) (-0.8846, 42.3202) (-0.9141, 42.3196) (-0.9435, 42.3189) (-0.9729, 42.318) (-1.0022, 42.3168) (-1.0315, 42.3155) (-1.0607, 42.314) (-1.0899, 42.3122) (-1.119, 42.3102) (-1.148, 42.308) (-1.177, 42.3055) (-1.2059, 42.3029) (-1.2347, 42.3) (-1.2635, 42.297) (-1.2922, 42.2937) (-1.3208, 42.2901) (-1.3493, 42.2863) (-1.3778, 42.2821) (-1.4061, 42.2776) (-1.4343, 42.2727) (-1.4624, 42.2675) (-1.4904, 42.262) (-1.5184, 42.2564) (-1.5462, 42.2506) (-1.574, 42.2445) (-1.6016, 42.238) (-1.629, 42.2307) (-1.6506, 42.224) (-1.6666, 42.2185) (-1.6772, 42.2145) (-1.6825, 42.2125) knots -1 -1 -1 -1 -1 -1 -0.98571429 -0.97142857 -0.95714286 -0.94285714 -0.92857143 -0.91428571 -0.9 -0.88571429 -0.87142857 -0.85714286 -0.84285714 -0.82857143 -0.81428571 -0.8 -0.78571429 -0.77142857 -0.75714286 -0.74285714 -0.72857143 -0.71428571 -0.7 -0.68571429 -0.67142857 -0.65714286 -0.64285714 -0.62857143 -0.61428571 -0.6 -0.58571429 -0.57142857 -0.55714286 -0.54285714 -0.52857143 -0.51428571 -0.5 -0.48571429 -0.47142857 -0.45714286 -0.44285714 -0.42857143 -0.41428571 -0.4 -0.38571429 -0.37142857 -0.35714286 -0.34285714 -0.32857143 -0.31428571 -0.3 -0.28571429 -0.27142857 -0.25714286 -0.24285714 -0.22857143 -0.21428571 -0.2 -0.18571429 -0.17142857 -0.15714286 -0.14285714 -0.12857143 -0.11428571 -0.1 -0.08571429 -0.07142857 -0.05714286 -0.04285714 -0.02857143 -0.01428571 0 0 0 0 0 0
  line L27 (-1.6825, 42.2125) -> (-2.1366, 42.0359)
  arc A55 (-2.2657, 42.092) -> (-2.1366, 42.0359) centre (-2.1728, 42.1291) ccw
  arc A56 (-2.2657, 42.092) -> (-2.6854, 43.0251) centre (-13.5, 37.5997) ccw
  arc A57 (-2.6417, 43.1589) -> (-2.6854, 43.0251) centre (-2.596, 43.0699) ccw
  line L28 (-2.6417, 43.1589) -> (-2.2083, 43.3815)
  spline S28 degree 5 poles (-2.2083, 43.3815) (-2.2033, 43.3841) (-2.1933, 43.3894) (-2.1785, 43.3977) (-2.1592, 43.4094) (-2.1356, 43.4251) (-2.1124, 43.4414) (-2.0894, 43.4582) (-2.0666, 43.4752) (-2.0438, 43.4924) (-2.0212, 43.5097) (-1.9986, 43.5273) (-1.9762, 43.5451) (-1.954, 43.5633) (-1.9321, 43.5818) (-1.9103, 43.6006) (-1.8886, 43.6197) (-1.8671, 43.639) (-1.8457, 43.6585) (-1.8245, 43.6781) (-1.8033, 43.698) (-1.7822, 43.718) (-1.7613, 43.7383) (-1.7405, 43.7587) (-1.7199, 43.7794) (-1.6993, 43.8002) (-1.6789, 43.8212) (-1.6586, 43.8424) (-1.6384, 43.8638) (-1.6184, 43.8853) (-1.5984, 43.907) (-1.5785, 43.9289) (-1.5588, 43.9509) (-1.5391, 43.9731) (-1.5196, 43.9954) (-1.5002, 44.0179) (-1.4809, 44.0406) (-1.4617, 44.0633) (-1.4426, 44.0863) (-1.4236, 44.1094) (-1.4047, 44.1326) (-1.3859, 44.156) (-1.3672, 44.1795) (-1.3486, 44.2031) (-1.3301, 44.2269) (-1.3117, 44.2508) (-1.2934, 44.2749) (-1.2752, 44.2991) (-1.2571, 44.3234) (-1.2392, 44.3479) (-1.2213, 44.3724) (-1.2035, 44.3972) (-1.1858, 44.422) (-1.1682, 44.4469) (-1.1507, 44.472) (-1.1333, 44.4972) (-1.116, 44.5226) (-1.0988, 44.548) (-1.0817, 44.5736) (-1.0647, 44.5992) (-1.0478, 44.625) (-1.031, 44.651) (-1.0143, 44.677) (-0.9977, 44.7031) (-0.9812, 44.7294) (-0.9647, 44.7558) (-0.9484, 44.7822) (-0.9322, 44.8088) (-0.916, 44.8355) (-0.9, 44.8624) (-0.884, 44.8893) (-0.8714, 44.9109) (-0.8619, 44.9272) (-0.8556, 44.938) (-0.8525, 44.9435) knots 0 0 0 0 0 0 0.01428571 0.02857143 0.04285714 0.05714286 0.07142857 0.08571429 0.1 0.11428571 0.12857143 0.14285714 0.15714286 0.17142857 0.18571429 0.2 0.21428571 0.22857143 0.24285714 0.25714286 0.27142857 0.28571429 0.3 0.31428571 0.32857143 0.34285714 0.35714286 0.37142857 0.38571429 0.4 0.41428571 0.42857143 0.44285714 0.45714286 0.47142857 0.48571429 0.5 0.51428571 0.52857143 0.54285714 0.55714286 0.57142857 0.58571429 0.6 0.61428571 0.62857143 0.64285714 0.65714286 0.67142857 0.68571429 0.7 0.71428571 0.72857143 0.74285714 0.75714286 0.77142857 0.78571429 0.8 0.81428571 0.82857143 0.84285714 0.85714286 0.87142857 0.88571429 0.9 0.91428571 0.92857143 0.94285714 0.95714286 0.97142857 0.98571429 1 1 1 1 1 1
  arc A58 (-0.8525, 44.9435) -> (-1.2756, 45.6281) centre (-13.5, 37.5997) ccw
  spline S29 degree 5 poles (-1.2756, 45.6281) (-1.2819, 45.6278) (-1.2944, 45.627) (-1.3132, 45.6258) (-1.3382, 45.6241) (-1.3694, 45.6219) (-1.4006, 45.6195) (-1.4317, 45.617) (-1.4627, 45.6144) (-1.4937, 45.6117) (-1.5246, 45.6088) (-1.5555, 45.6057) (-1.5863, 45.6026) (-1.6171, 45.5992) (-1.6478, 45.5958) (-1.6784, 45.5922) (-1.709, 45.5885) (-1.7395, 45.5846) (-1.77, 45.5806) (-1.8004, 45.5765) (-1.8307, 45.5722) (-1.8609, 45.5678) (-1.8911, 45.5632) (-1.9212, 45.5585) (-1.9513, 45.5536) (-1.9813, 45.5486) (-2.0112, 45.5434) (-2.041, 45.5381) (-2.0708, 45.5327) (-2.1005, 45.5271) (-2.1301, 45.5214) (-2.1597, 45.5155) (-2.1891, 45.5094) (-2.2185, 45.5032) (-2.2478, 45.4968) (-2.2771, 45.4903) (-2.3062, 45.4836) (-2.3353, 45.4768) (-2.3642, 45.4698) (-2.3931, 45.4627) (-2.4219, 45.4554) (-2.4507, 45.4479) (-2.4793, 45.4402) (-2.5078, 45.4324) (-2.5362, 45.4244) (-2.5646, 45.4163) (-2.5928, 45.4079) (-2.6209, 45.3994) (-2.649, 45.3908) (-2.6769, 45.3819) (-2.7047, 45.3729) (-2.7324, 45.3636) (-2.76, 45.3542) (-2.7875, 45.3445) (-2.8148, 45.3346) (-2.842, 45.3246) (-2.8692, 45.3144) (-2.8962, 45.3039) (-2.923, 45.2933) (-2.9498, 45.2825) (-2.9763, 45.2714) (-3.0027, 45.26) (-3.0289, 45.2483) (-3.0549, 45.2363) (-3.0807, 45.224) (-3.1063, 45.2115) (-3.1319, 45.1988) (-3.1573, 45.186) (-3.1826, 45.1729) (-3.2075, 45.1595) (-3.2321, 45.1453) (-3.2512, 45.1333) (-3.2653, 45.1238) (-3.2745, 45.1172) (-3.279, 45.1139) knots -1 -1 -1 -1 -1 -1 -0.98571429 -0.97142857 -0.95714286 -0.94285714 -0.92857143 -0.91428571 -0.9 -0.88571429 -0.87142857 -0.85714286 -0.84285714 -0.82857143 -0.81428571 -0.8 -0.78571429 -0.77142857 -0.75714286 -0.74285714 -0.72857143 -0.71428571 -0.7 -0.68571429 -0.67142857 -0.65714286 -0.64285714 -0.62857143 -0.61428571 -0.6 -0.58571429 -0.57142857 -0.55714286 -0.54285714 -0.52857143 -0.51428571 -0.5 -0.48571429 -0.47142857 -0.45714286 -0.44285714 -0.42857143 -0.41428571 -0.4 -0.38571429 -0.37142857 -0.35714286 -0.34285714 -0.32857143 -0.31428571 -0.3 -0.28571429 -0.27142857 -0.25714286 -0.24285714 -0.22857143 -0.21428571 -0.2 -0.18571429 -0.17142857 -0.15714286 -0.14285714 -0.12857143 -0.11428571 -0.1 -0.08571429 -0.07142857 -0.05714286 -0.04285714 -0.02857143 -0.01428571 0 0 0 0 0 0
  line L29 (-3.279, 45.1139) -> (-3.672, 44.8258)
  arc A59 (-3.8112, 44.8466) -> (-3.672, 44.8258) centre (-3.7311, 44.9065) ccw
  arc A60 (-3.8112, 44.8466) -> (-4.4581, 45.6393) centre (-13.5, 37.5997) ccw
  arc A61 (-4.4505, 45.7798) -> (-4.4581, 45.6393) centre (-4.3833, 45.7057) ccw
  line L30 (-4.4505, 45.7798) -> (-4.0895, 46.107)
  spline S30 degree 5 poles (-4.0895, 46.107) (-4.0853, 46.1108) (-4.0771, 46.1185) (-4.0649, 46.1303) (-4.0493, 46.1467) (-4.0305, 46.1679) (-4.0124, 46.1897) (-3.9945, 46.2118) (-3.9768, 46.2342) (-3.9593, 46.2566) (-3.9419, 46.2793) (-3.9247, 46.3021) (-3.9077, 46.3251) (-3.891, 46.3484) (-3.8745, 46.372) (-3.8583, 46.3958) (-3.8423, 46.4198) (-3.8266, 46.444) (-3.811, 46.4684) (-3.7955, 46.4929) (-3.7802, 46.5175) (-3.7651, 46.5423) (-3.7501, 46.5673) (-3.7353, 46.5924) (-3.7207, 46.6177) (-3.7062, 46.6432) (-3.692, 46.6688) (-3.6778, 46.6945) (-3.6639, 46.7204) (-3.6501, 46.7464) (-3.6364, 46.7725) (-3.6229, 46.7987) (-3.6095, 46.8251) (-3.5962, 46.8516) (-3.5832, 46.8782) (-3.5702, 46.905) (-3.5574, 46.9319) (-3.5448, 46.9589) (-3.5323, 46.986) (-3.5199, 47.0132) (-3.5076, 47.0405) (-3.4955, 47.0679) (-3.4836, 47.0955) (-3.4717, 47.1232) (-3.46, 47.1509) (-3.4485, 47.1788) (-3.437, 47.2068) (-3.4257, 47.2348) (-3.4145, 47.263) (-3.4035, 47.2913) (-3.3926, 47.3196) (-3.3818, 47.3481) (-3.3711, 47.3767) (-3.3606, 47.4053) (-3.3502, 47.4341) (-3.3399, 47.4629) (-3.3298, 47.4919) (-3.3197, 47.5209) (-3.3098, 47.55) (-3.3001, 47.5792) (-3.2904, 47.6085) (-3.2809, 47.6379) (-3.2715, 47.6674) (-3.2622, 47.6969) (-3.253, 47.7266) (-3.244, 47.7563) (-3.2351, 47.7861) (-3.2263, 47.816) (-3.2176, 47.846) (-3.209, 47.876) (-3.2006, 47.9061) (-3.1939, 47.9303) (-3.189, 47.9485) (-3.1857, 47.9606) (-3.1841, 47.9666) knots 0 0 0 0 0 0 0.01428571 0.02857143 0.04285714 0.05714286 0.07142857 0.08571429 0.1 0.11428571 0.12857143 0.14285714 0.15714286 0.17142857 0.18571429 0.2 0.21428571 0.22857143 0.24285714 0.25714286 0.27142857 0.28571429 0.3 0.31428571 0.32857143 0.34285714 0.35714286 0.37142857 0.38571429 0.4 0.41428571 0.42857143 0.44285714 0.45714286 0.47142857 0.48571429 0.5 0.51428571 0.52857143 0.54285714 0.55714286 0.57142857 0.58571429 0.6 0.61428571 0.62857143 0.64285714 0.65714286 0.67142857 0.68571429 0.7 0.71428571 0.72857143 0.74285714 0.75714286 0.77142857 0.78571429 0.8 0.81428571 0.82857143 0.84285714 0.85714286 0.87142857 0.88571429 0.9 0.91428571 0.92857143 0.94285714 0.95714286 0.97142857 0.98571429 1 1 1 1 1 1
  arc A62 (-3.1841, 47.9666) -> (-3.7701, 48.5185) centre (-13.5, 37.5997) ccw
  spline S31 degree 5 poles (-3.7701, 48.5185) (-3.776, 48.5165) (-3.7879, 48.5125) (-3.8058, 48.5065) (-3.8295, 48.4984) (-3.8591, 48.4882) (-3.8885, 48.4778) (-3.9179, 48.4674) (-3.9472, 48.4568) (-3.9765, 48.4461) (-4.0056, 48.4353) (-4.0346, 48.4244) (-4.0636, 48.4133) (-4.0924, 48.4022) (-4.1212, 48.3909) (-4.1498, 48.3795) (-4.1784, 48.368) (-4.2069, 48.3564) (-4.2353, 48.3446) (-4.2635, 48.3328) (-4.2917, 48.3208) (-4.3198, 48.3087) (-4.3478, 48.2964) (-4.3757, 48.2841) (-4.4034, 48.2716) (-4.4311, 48.259) (-4.4587, 48.2463) (-4.4861, 48.2334) (-4.5134, 48.2205) (-4.5407, 48.2074) (-4.5678, 48.1942) (-4.5948, 48.1808) (-4.6217, 48.1674) (-4.6485, 48.1538) (-4.6752, 48.14) (-4.7017, 48.1262) (-4.7281, 48.1122) (-4.7544, 48.0981) (-4.7806, 48.0838) (-4.8067, 48.0694) (-4.8326, 48.0549) (-4.8584, 48.0402) (-4.8841, 48.0255) (-4.9096, 48.0105) (-4.935, 47.9954) (-4.9602, 47.9802) (-4.9854, 47.9649) (-5.0103, 47.9494) (-5.0352, 47.9337) (-5.0599, 47.918) (-5.0844, 47.902) (-5.1088, 47.8859) (-5.133, 47.8696) (-5.157, 47.8532) (-5.1809, 47.8366) (-5.2046, 47.8199) (-5.2281, 47.803) (-5.2515, 47.7859) (-5.2747, 47.7687) (-5.2977, 47.7513) (-5.3205, 47.7337) (-5.3431, 47.7159) (-5.3653, 47.6978) (-5.3873, 47.6795) (-5.409, 47.6609) (-5.4305, 47.6422) (-5.4519, 47.6233) (-5.4732, 47.6044) (-5.4942, 47.5852) (-5.5149, 47.5657) (-5.5349, 47.5458) (-5.5503, 47.5292) (-5.5614, 47.5164) (-5.5686, 47.5076) (-5.5721, 47.5032) knots -1 -1 -1 -1 -1 -1 -0.98571429 -0.97142857 -0.95714286 -0.94285714 -0.92857143 -0.91428571 -0.9 -0.88571429 -0.87142857 -0.85714286 -0.84285714 -0.82857143 -0.81428571 -0.8 -0.78571429 -0.77142857 -0.75714286 -0.74285714 -0.72857143 -0.71428571 -0.7 -0.68571429 -0.67142857 -0.65714286 -0.64285714 -0.62857143 -0.61428571 -0.6 -0.58571429 -0.57142857 -0.55714286 -0.54285714 -0.52857143 -0.51428571 -0.5 -0.48571429 -0.47142857 -0.45714286 -0.44285714 -0.42857143 -0.41428571 -0.4 -0.38571429 -0.37142857 -0.35714286 -0.34285714 -0.32857143 -0.31428571 -0.3 -0.28571429 -0.27142857 -0.25714286 -0.24285714 -0.22857143 -0.21428571 -0.2 -0.18571429 -0.17142857 -0.15714286 -0.14285714 -0.12857143 -0.11428571 -0.1 -0.08571429 -0.07142857 -0.05714286 -0.04285714 -0.02857143 -0.01428571 0 0 0 0 0 0
  line L31 (-5.5721, 47.5032) -> (-5.8771, 47.1233)
  arc A63 (-6.0169, 47.1073) -> (-5.8771, 47.1233) centre (-5.9551, 47.1859) ccw
  arc A64 (-6.0169, 47.1073) -> (-6.847, 47.7055) centre (-13.5, 37.5997) ccw
  arc A65 (-6.876, 47.8432) -> (-6.847, 47.7055) centre (-6.792, 47.7891) ccw
  line L32 (-6.876, 47.8432) -> (-6.612, 48.2527)
  spline S32 degree 5 poles (-6.612, 48.2527) (-6.609, 48.2575) (-6.603, 48.2671) (-6.5943, 48.2816) (-6.5834, 48.3015) (-6.5708, 48.3268) (-6.5589, 48.3526) (-6.5474, 48.3786) (-6.5361, 48.4047) (-6.525, 48.431) (-6.514, 48.4573) (-6.5033, 48.4838) (-6.4928, 48.5105) (-6.4827, 48.5373) (-6.4729, 48.5643) (-6.4634, 48.5915) (-6.4542, 48.6188) (-6.4453, 48.6463) (-6.4365, 48.6739) (-6.4279, 48.7016) (-6.4195, 48.7293) (-6.4113, 48.7572) (-6.4033, 48.7852) (-6.3955, 48.8133) (-6.3879, 48.8415) (-6.3806, 48.8698) (-6.3734, 48.8982) (-6.3664, 48.9268) (-6.3596, 48.9554) (-6.353, 48.984) (-6.3466, 49.0128) (-6.3403, 49.0417) (-6.3342, 49.0706) (-6.3283, 49.0996) (-6.3225, 49.1287) (-6.317, 49.1579) (-6.3116, 49.1872) (-6.3063, 49.2166) (-6.3012, 49.246) (-6.2963, 49.2755) (-6.2916, 49.305) (-6.287, 49.3347) (-6.2825, 49.3644) (-6.2783, 49.3942) (-6.2742, 49.424) (-6.2702, 49.4539) (-6.2664, 49.4839) (-6.2627, 49.5139) (-6.2592, 49.544) (-6.2559, 49.5742) (-6.2527, 49.6044) (-6.2496, 49.6347) (-6.2467, 49.6651) (-6.244, 49.6955) (-6.2414, 49.726) (-6.2389, 49.7565) (-6.2366, 49.7871) (-6.2344, 49.8177) (-6.2324, 49.8484) (-6.2305, 49.8791) (-6.2288, 49.9099) (-6.2272, 49.9408) (-6.2257, 49.9717) (-6.2244, 50.0026) (-6.2232, 50.0336) (-6.2222, 50.0647) (-6.2213, 50.0958) (-6.2205, 50.1269) (-6.2199, 50.1581) (-6.2194, 50.1893) (-6.219, 50.2206) (-6.2189, 50.2457) (-6.2188, 50.2645) (-6.2188, 50.2771) (-6.2188, 50.2833) knots 0 0 0 0 0 0 0.01428571 0.02857143 0.04285714 0.05714286 0.07142857 0.08571429 0.1 0.11428571 0.12857143 0.14285714 0.15714286 0.17142857 0.18571429 0.2 0.21428571 0.22857143 0.24285714 0.25714286 0.27142857 0.28571429 0.3 0.31428571 0.32857143 0.34285714 0.35714286 0.37142857 0.38571429 0.4 0.41428571 0.42857143 0.44285714 0.45714286 0.47142857 0.48571429 0.5 0.51428571 0.52857143 0.54285714 0.55714286 0.57142857 0.58571429 0.6 0.61428571 0.62857143 0.64285714 0.65714286 0.67142857 0.68571429 0.7 0.71428571 0.72857143 0.74285714 0.75714286 0.77142857 0.78571429 0.8 0.81428571 0.82857143 0.84285714 0.85714286 0.87142857 0.88571429 0.9 0.91428571 0.92857143 0.94285714 0.95714286 0.97142857 0.98571429 1 1 1 1 1 1
  arc A66 (-6.2188, 50.2833) -> (-6.9276, 50.6647) centre (-13.5, 37.5997) ccw
  spline S33 degree 5 poles (-6.9276, 50.6647) (-6.9328, 50.6613) (-6.9433, 50.6543) (-6.959, 50.6439) (-6.9798, 50.6299) (-7.0057, 50.6124) (-7.0315, 50.5948) (-7.0572, 50.5771) (-7.0828, 50.5593) (-7.1082, 50.5414) (-7.1336, 50.5234) (-7.1588, 50.5054) (-7.1839, 50.4872) (-7.2089, 50.469) (-7.2337, 50.4506) (-7.2585, 50.4322) (-7.2831, 50.4137) (-7.3076, 50.3951) (-7.3319, 50.3764) (-7.3562, 50.3576) (-7.3803, 50.3387) (-7.4043, 50.3198) (-7.4281, 50.3007) (-7.4519, 50.2816) (-7.4755, 50.2623) (-7.4989, 50.243) (-7.5223, 50.2236) (-7.5455, 50.2041) (-7.5685, 50.1845) (-7.5914, 50.1648) (-7.6142, 50.145) (-7.6368, 50.1251) (-7.6593, 50.1051) (-7.6817, 50.0851) (-7.7039, 50.0649) (-7.7259, 50.0447) (-7.7479, 50.0243) (-7.7696, 50.0039) (-7.7912, 49.9833) (-7.8127, 49.9627) (-7.8339, 49.9419) (-7.8551, 49.9211) (-7.876, 49.9002) (-7.8968, 49.8791) (-7.9174, 49.858) (-7.9379, 49.8368) (-7.9582, 49.8154) (-7.9783, 49.794) (-7.9983, 49.7725) (-8.018, 49.7508) (-8.0376, 49.7291) (-8.057, 49.7072) (-8.0761, 49.6852) (-8.0951, 49.6632) (-8.1138, 49.6409) (-8.1324, 49.6186) (-8.1507, 49.5962) (-8.1689, 49.5737) (-8.1869, 49.5511) (-8.2046, 49.5283) (-8.2221, 49.5054) (-8.2393, 49.4824) (-8.2561, 49.4591) (-8.2725, 49.4357) (-8.2887, 49.4122) (-8.3047, 49.3885) (-8.3205, 49.3648) (-8.3361, 49.341) (-8.3514, 49.317) (-8.3663, 49.2929) (-8.3805, 49.2684) (-8.3911, 49.2484) (-8.3985, 49.2331) (-8.4032, 49.2228) (-8.4055, 49.2177) knots -1 -1 -1 -1 -1 -1 -0.98571429 -0.97142857 -0.95714286 -0.94285714 -0.92857143 -0.91428571 -0.9 -0.88571429 -0.87142857 -0.85714286 -0.84285714 -0.82857143 -0.81428571 -0.8 -0.78571429 -0.77142857 -0.75714286 -0.74285714 -0.72857143 -0.71428571 -0.7 -0.68571429 -0.67142857 -0.65714286 -0.64285714 -0.62857143 -0.61428571 -0.6 -0.58571429 -0.57142857 -0.55714286 -0.54285714 -0.52857143 -0.51428571 -0.5 -0.48571429 -0.47142857 -0.45714286 -0.44285714 -0.42857143 -0.41428571 -0.4 -0.38571429 -0.37142857 -0.35714286 -0.34285714 -0.32857143 -0.31428571 -0.3 -0.28571429 -0.27142857 -0.25714286 -0.24285714 -0.22857143 -0.21428571 -0.2 -0.18571429 -0.17142857 -0.15714286 -0.14285714 -0.12857143 -0.11428571 -0.1 -0.08571429 -0.07142857 -0.05714286 -0.04285714 -0.02857143 -0.01428571 0 0 0 0 0 0
  line L33 (-8.4055, 49.2177) -> (-8.6017, 48.7717)
  arc A67 (-8.7326, 48.7201) -> (-8.6017, 48.7717) centre (-8.6932, 48.812) ccw
  arc A68 (-8.7326, 48.7201) -> (-9.6892, 49.0831) centre (-13.5, 37.5997) ccw
  arc A69 (-9.7529, 49.2086) -> (-9.6892, 49.0831) centre (-9.6577, 49.178) ccw
  line L34 (-9.7529, 49.2086) -> (-9.6039, 49.6725)